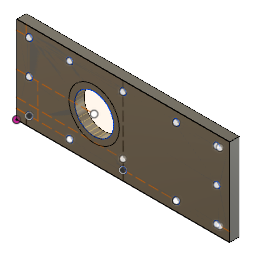
sidepanel v16 (Autodesk Fusion 360 design; units mm, degrees)
Autodesk Fusion 360 part; units mm, degrees
sketch "Sketch1" plane through (0, 0, 0) normal (0, 0, 1) x (1, 0, 0)
  line L0 (0, 0) -> (139.7, 0)
  line L1 (139.7, 0) -> (139.7, 57.15)
  line L2 (139.7, 57.15) -> (0, 57.15)
  line L3 (0, 57.15) -> (0, 0)
  line L4 (0, 28.575) -> (50.8, 28.575) construction
  circle A0 centre (50.8, 28.575) radius 12.7
  line L5 (0, 12.7) -> (69.85, 12.7) construction
  line L6 (69.85, 0) -> (69.85, 57.15) construction
  line L7 (0, 6.35) -> (6.35, 6.35) construction
  line L8 (6.35, 0) -> (6.35, 6.35) construction
  circle A1 centre (8.3337, 6.35) radius 1.9837
  circle A2 centre (69.85, 6.35) radius 1.9837
  line L9 (0, 6.35) -> (34.925, 6.35) construction
  circle A3 centre (34.925, 6.35) radius 1.9837
  line L10 (69.85, 6.35) -> (104.775, 6.35) construction
  circle A4 centre (104.775, 6.35) radius 1.9837
  line L11 (139.7, 6.3229) -> (133.35, 6.3229) construction
  circle A5 centre (131.3688, 6.35) radius 1.9837
  circle A6 centre (8.3337, 50.8) radius 1.9837
  circle A7 centre (34.925, 50.8) radius 1.9837
  circle A8 centre (69.85, 50.8) radius 1.9837
  circle A9 centre (104.775, 50.8) radius 1.9837
  circle A10 centre (131.3688, 50.8) radius 1.9837
  line L12 (0, 50.8) -> (6.35, 50.8) construction
  line L13 (6.35, 57.15) -> (6.35, 50.8) construction
  line L14 (13.97, 6.35) -> (13.97, 28.575) construction
  circle A11 centre (8.3337, 28.575) radius 1.9837
  circle A12 centre (131.3688, 28.575) radius 1.9837
  point P0 (8.3337, 6.35)
  point P1 (8.3337, 6.35)
  point P2 (133.35, 50.7729)
  dimension "d1" = 57.15
  dimension "d2" = 139.7
  dimension "d28" = 25.4
  dimension "d33" = 1.9837
  dimension "d34" = 6.35
  dimension "d35" = 34.925
  dimension "d36" = 34.925
  dimension "d37" = 6.35
  measures "d1" distance of L0.start L2.end
  measures "d2" distance of L0.start L0.end
  measures "d28" diameter of A0
  measures "d33" distance of L7.end P1
  measures "d34" distance of L7.start L7.end
  measures "d35" distance of L7.start L9.end
  measures "d36" distance of A2.centre L10.end
  measures "d37" distance of L11.start L11.end
surface "Extrude4" add extruded along (0, 0, 1) between 0 and -6.35 profiles "Sketch1" section 1 makes body 1 at (93.1333, 57.15, -2.1167) makes body 2 at (34.8755, 52.7831, -4.2333) makes body 3 at (10.3076, 50.6025, -4.2333) makes body 4 at (131.7133, 30.5286, -4.2333) makes body 5 at (63.4369, 27.3105, -4.2333) makes body 6 at (71.2351, 7.7701, -4.2333) makes body 7 at (106.1601, 7.7701, -4.2333) makes body 8 at (131.7133, 52.7536, -4.2333) makes body 9 at (10.3076, 6.1525, -4.2333) makes body 10 at (34.8755, 8.3331, -4.2333) makes body 11 at (106.1601, 52.2201, -4.2333) makes body 12 at (131.6155, 4.3817, -2.1167) makes body 13 at (10.3076, 28.3775, -4.2333) makes body 14 at (71.2351, 52.2201, -4.2333)
extrude "Extrude3" add sketch "Sketch1" against normal blind 6.35 separate body contours L0 L1 L2 L3 | A1 | A2 | A3 | A4 | A5 | A6 | A7 | A8 | A9 | A10 | A11 | A12 makes body 15
extrude "Extrude2" add sketch "Sketch1" against normal blind 6.35 separate body contours L0 L1 L2 L3 | A1 | A2 | A3 | A4 | A5 | A6 | A7 | A8 | A9 | A10 | A11 | A12 makes body 16
sketch "Sketch2" plane through (0, 0, 0) normal (0, 0, 1) x (1, 0, 0)
  line L0 (0, 57.15) -> (0, 0)
  line L1 (0, 28.575) -> (50.8, 28.575) construction
  circle A0 centre (50.8, 28.575) radius 12.7
  point P0 (50.8, 28.575)
  dimension "d22" = 25.4
  measures "d22" diameter of A0
extrude "Extrude1" add sketch "Sketch1" against normal blind 6.35 separate body contours L0 L1 L2 L3 | A0 | A1 | A2 | A3 | A4 | A5 | A6 | A7 | A8 | A9 | A10 | A11 | A12 makes body 17
hole "Hole1" at (50.8, 28.575, 0) direction (0, 0, -1) diameter 33.02 depth 33.02 tip angle 118 bodies 17
